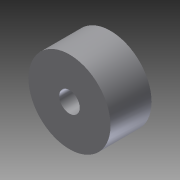
# Autodesk Inventor part: magnet_125
Saved by Autodesk Inventor 2011 (Build 150239000, 239)
## iProperties
Created: 2012-06-13
Part Number: magnet_125
Document SubType Name: Modeling
Designer: labuser
Density: 1 g/cm^3
Author: labuser
Autodesk Inventor part; units mm, degrees
ref_plane "YZ Plane" through (0, 0, 0) normal (1, 0, 0) x (0, 1, 0)
ref_plane "XZ Plane" through (0, 0, 0) normal (0, 1, 0) x (-1, 0, 0)
ref_plane "XY Plane" through (0, 0, 0) normal (0, 0, 1) x (1, 0, 0)
sketch "Sketch1" plane through (0, 0, 0) normal (0, 0, 1) x (1, 0, 0)
  circle A0 centre (0, 0) radius 6.35
  circle A1 centre (0, 0) radius 1.5875
  dimension "d1" = 12.7
  dimension "d2" = 3.175
  constraints: 2 centre point, 2 coincident
  measures "d1" diameter of A0
  measures "d2" diameter of A1
extrude "Extrusion1" add sketch "Sketch1" along normal blind 6.35
body "Solid1"
